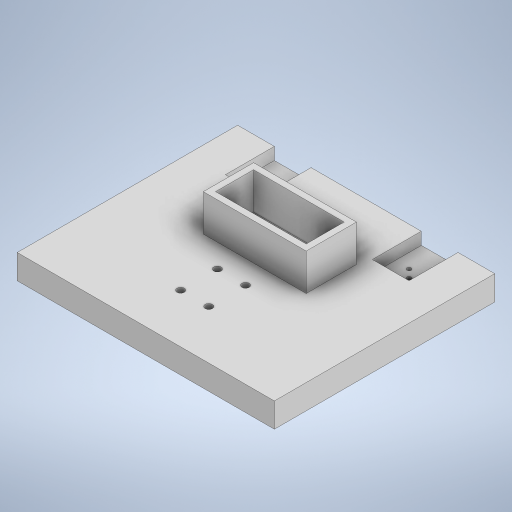
# Autodesk Inventor part: base_front
Saved by Autodesk Inventor 2023 (Build 270158000, 158)
## iProperties
Created: 2022-10-20
Part Number: base_front
Material: Genérico
Document SubType Name: Modeling
Designer: inigo
Density: 1 g/cm^3
Appearance: Valor por defecto
Author: inigo
Autodesk Inventor part; units mm, degrees
ref_plane "YZ Plane" through (0, 0, 0) normal (1, 0, 0) x (0, 1, 0)
ref_plane "XZ Plane" through (0, 0, 0) normal (0, 1, 0) x (-1, 0, 0)
ref_plane "XY Plane" through (0, 0, 0) normal (0, 0, 1) x (1, 0, 0)
sketch "Boceto1" plane through (0, 0, 0) normal (0, 1, 0) x (-1, 0, 0)
  line L0 (105, 90) -> (-105, 90)
  line L1 (-105, 90) -> (-105, -90)
  line L2 (-105, -90) -> (105, -90)
  line L3 (105, -90) -> (105, 90)
  line L4 (105, 90) -> (-105, -90) construction
  line L5 (-105, 90) -> (105, -90) construction
  point P0 (0, 0)
  dimension "d0" = 210
  dimension "d1" = 180
  constraints: 12 end point, 2 midpoint, 2 parallel, 1 horizontal, 1 perpendicular
  measures "d0" distance of L2.end L1.end
  measures "d1" distance of L1.end L0.end
extrude "Extrusión1" add sketch "Boceto1" along normal blind 20
sketch "Boceto2" plane through (0, 20, 0) normal (0, 1, 0) x (1, 0, 0)
  line L0 (-105.0239, -70) -> (104.9761, -70)
  line L1 (-105.0239, -70) -> (104.9761, -70)
  circle A0 centre (-11.5239, -50) radius 3
  circle A1 centre (11.4761, -50) radius 3
  circle A2 centre (-11.5239, -20) radius 3
  circle A3 centre (11.4761, -20) radius 3
  line L2 (-105, -90) -> (105, -90) projected
  circle A4 centre (28, 59) radius 3.5
  circle A5 centre (-28, 59) radius 3.5
  line L3 (105, 90) -> (-105, 90) projected
  line L4 (0, 90) -> (0, 53.0386)
  point P0 (0, 0)
  point P1 (0, -225)
  point P2 (0, -225)
  dimension "d4" = 20
  dimension "d5" = 20
  dimension "d6" = 30
  dimension "d7" = 30
  dimension "d8" = 20
  dimension "d9" = 7
  dimension "d11" = 7
  dimension "d12" = 31
  dimension "d13" = 31
  dimension "d14" = 28
  dimension "d15" = 28
  constraints: 6 centre point, 6 end point, 1 collinear, 1 midpoint, 1 vertical
  measures "d4" distance from line of L0 A0.centre
  measures "d5" distance from line of A1.centre L0
  measures "d6" distance between centres of A3 A1
  measures "d7" distance of A2.centre A0.centre
  measures "d8" distance between parallel lines of L2 L0
  measures "d9" diameter of A4
  measures "d11" diameter of A5
  measures "d12" distance from line of A5.centre L3
  measures "d13" distance from line of L3 A4.centre
  measures "d14" distance from line of L4 A4.centre
  measures "d15" distance from line of L4 A5.centre
extrude "Extrusión2" cut sketch "Boceto2" against normal blind 20 contours A0 | A1 | A2 | A3
sketch "Boceto3" plane through (0, 20, 0) normal (0, 1, 0) x (1, 0, 0)
  line L0 (105, 90) -> (-105, 90) projected
  line L1 (0, 90) -> (0, 58.0056)
  circle A0 centre (-28, 59) radius 3.5 projected
  line L2 (-42, -1) -> (42, -1)
  line L3 (42, -1) -> (42, 40)
  line L4 (42, 40) -> (-42, 40)
  line L5 (-42, 40) -> (-42, -1)
  line L6 (-42, -1) -> (42, 40) construction
  line L7 (42, -1) -> (-42, 40) construction
  circle A1 centre (-11.5239, -20) radius 3 projected
  line L8 (-37, 4) -> (37, 4)
  line L9 (37, 4) -> (37, 35)
  line L10 (37, 35) -> (-37, 35)
  line L11 (-37, 35) -> (-37, 4)
  line L12 (-37, 4) -> (37, 35) construction
  line L13 (37, 4) -> (-37, 35) construction
  point P0 (0, 0)
  point P1 (-24.876, 34.9118)
  point P2 (0, 74.0028)
  point P3 (0, 19.5)
  dimension "d23" = 84
  dimension "d24" = 41
  dimension "d25" = 19
  dimension "d26" = 74
  dimension "d27" = 31
  constraints: 26 end point, 6 midpoint, 4 parallel, 2 horizontal, 2 perpendicular, 1 vertical
  measures "d23" distance of L4.end L3.end
  measures "d24" distance of L3.end L2.end
  measures "d25" distance from line of L2 A1.centre
  measures "d26" distance of L10.end L9.end
  measures "d27" distance of L9.end L8.end
extrude "Extrusión3" add sketch "Boceto3" along normal blind 30 contours L5 L4 L3 L2
sketch "Boceto4" plane through (0, 20, 0) normal (0, 1, 0) x (1, 0, 0)
  circle A0 centre (-56.75, 68.25) radius 1.75
  line L0 (105, 90) -> (-105, 90) projected
  line L1 (-55, 60) -> (-65, 60)
  line L2 (-65, 60) -> (-65, 70)
  line L3 (-65, 70) -> (-55, 70)
  line L4 (-55, 70) -> (-55, 60)
  line L5 (-55, 60) -> (-65, 70) construction
  line L6 (-65, 60) -> (-55, 70) construction
  line L7 (-105, 90) -> (-105, -90) projected
  circle A1 centre (-63.25, 61.75) radius 1.75
  line L8 (0, 90) -> (0, 77.3124)
  circle A2 centre (56.75, 68.25) radius 1.75
  line L9 (55, 60) -> (65, 60)
  line L10 (65, 60) -> (65, 70)
  line L11 (65, 70) -> (55, 70)
  line L12 (55, 70) -> (55, 60)
  line L13 (55, 60) -> (65, 70) construction
  line L14 (65, 60) -> (55, 70) construction
  circle A3 centre (63.25, 61.75) radius 1.75
  point P0 (0, 0)
  point P1 (-65, 65)
  point P2 (65, 65)
  dimension "d30" = 3.5
  dimension "d32" = 40
  dimension "d33" = 1.75
  dimension "d34" = 1.75
  dimension "d35" = 1.75
  dimension "d36" = 1.75
  dimension "d37" = 10
  dimension "d38" = 10
  dimension "d39" = 20
  constraints: 26 end point, 7 symmetric about line, 4 centre point, 2 midpoint, 2 parallel, 1 horizontal, 1 perpendicular, 1 vertical, 2 other
  measures "d30" diameter of A0
  measures "d32" distance from line of point (-65, 65) L7
  measures "d33" distance from line of L3 A0.centre
  measures "d34" distance from line of L4 A0.centre
  measures "d35" distance from line of L2 A1.centre
  measures "d36" distance from line of L1 A1.centre
  measures "d37" distance between parallel lines of L1 L3
  measures "d38" distance between parallel lines of L4 L2
  measures "d39" distance between parallel lines of L0 L3
hole "Agujero1" at (-63.25, 20, -61.75) at (-56.75, 20, -68.25) at (56.75, 20, -68.25) at (63.25, 20, -61.75) direction (0, -1, 0) diameter 3.5 end through all
sketch "Boceto5" plane through (0, 20, 0) normal (0, 1, 0) x (1, 0, 0)
  circle A0 centre (56.75, 68.25) radius 1.75 projected
  line L0 (55, 68.25) -> (55, 90.0503)
  circle A1 centre (63.25, 61.75) radius 1.75 projected
  line L1 (65, 61.75) -> (65, 90)
  line L2 (105, 90) -> (-105, 90) projected
  line L3 (55, 90.0503) -> (45.0001, 90)
  line L4 (65, 90) -> (75, 90)
  line L5 (45.0001, 90) -> (75, 90)
  line L6 (75, 90) -> (75, 50)
  line L7 (75, 50) -> (45.0001, 50)
  line L8 (45.0001, 50) -> (45.0001, 90)
  line L9 (0, 90) -> (0, 68.25)
  circle A2 centre (-56.75, 68.25) radius 1.75
  line L10 (-55, 68.25) -> (-55, 90.0503)
  circle A3 centre (-63.25, 61.75) radius 1.75
  line L11 (-65, 61.75) -> (-65, 90)
  line L12 (-105, 90) -> (105, 90)
  line L13 (-55, 90.0503) -> (-45.0001, 90)
  line L14 (-65, 90) -> (-75, 90)
  line L15 (-45.0001, 90) -> (-75, 90)
  line L16 (-75, 90) -> (-75, 50)
  line L17 (-75, 50) -> (-45.0001, 50)
  line L18 (-45.0001, 50) -> (-45.0001, 90)
  point P0 (0, 0)
  dimension "d47" = 10
  dimension "d48" = 10
  dimension "d49" = 40
  constraints: 36 end point, 13 symmetric about line, 6 point on line, 6 vertical, 4 horizontal alignment, 2 parallel, 1 horizontal, 1 midpoint, 1 perpendicular, 6 other
  measures "d47" distance of L0.end L3.end
  measures "d48" distance of L1.end L4.end
  measures "d49" distance of L5.end L6.end
extrude "Extrusión4" cut sketch "Boceto5" against normal blind 10 contours A0 | L2 L6 L7 L8 | A1 | L2 L18 L17 L16
